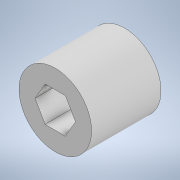
# Autodesk Inventor part: Climber Axel Spacer
Saved by Autodesk Inventor 2020 (Build 240168000, 168)
## iProperties
Created: 2020-02-03
Part Number: Climber Axel Spacer
Material: Generic
Document SubType Name: Modeling
Designer: JimAndVal
Density: 1 g/cm^3
Appearance: Default
Author: JimAndVal
Autodesk Inventor part; units mm, degrees
ref_plane "YZ Plane" through (0, 0, 0) normal (1, 0, 0) x (0, 1, 0)
ref_plane "XZ Plane" through (0, 0, 0) normal (0, 1, 0) x (-1, 0, 0)
ref_plane "XY Plane" through (0, 0, 0) normal (0, 0, 1) x (1, 0, 0)
sketch "Sketch1" plane through (0, 0, 0) normal (0, 0, 1) x (1, 0, 0)
  circle A0 centre (0, 0) radius 13.2715
  dimension "d0" = 26.543
  constraints: 1 centre point, 1 coincident
  measures "d0" diameter of A0
extrude "Extrusion1" add sketch "Sketch1" along normal mid plane 25.4
sketch "Sketch2" plane through (0, 0, 12.7) normal (0, 0, 1) x (1, 0, 0)
  circle A0 centre (0, 0) radius 6.4135 construction
  line L0 (3.6753, -6.4293) -> (-3.7303, -6.3976)
  line L1 (-3.7303, -6.3976) -> (-7.4056, 0.0317)
  line L2 (-7.4056, 0.0317) -> (-3.6753, 6.4293)
  line L3 (-3.6753, 6.4293) -> (3.7303, 6.3976)
  line L4 (3.7303, 6.3976) -> (7.4056, -0.0317)
  line L5 (7.4056, -0.0317) -> (3.6753, -6.4293)
  point P0 (5.5405, -3.2305)
  dimension "d3" = 12.827
  constraints: 12 end point, 2 coincident, 1 midpoint, 16 other
extrude "Extrusion2" cut sketch "Sketch2" against normal through all
body "Solid1"
